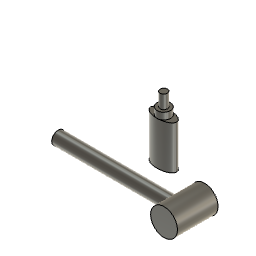
Part3, Assembly of Parts (Autodesk Fusion 360 design; units mm, degrees)
Autodesk Fusion 360 part; units mm, degrees
sketch "Sketch1" plane through (0, 0, 0) normal (0, 0, 1) x (1, 0, 0)
  ellipse E0 centre (0, 0) end of major axis (30.02, 0) minor radius 15.29
  line L0 (-30.02, 0) -> (30.02, 0) construction
  line L1 (0, -15.29) -> (0, 15.29) construction
  dimension "d1" = 60.04
  dimension "d2" = 30.58
  constraint coincident E0 L0.start
  constraint coincident E0 L0.end
  constraint coincident E0 L1.start
  constraint coincident E0 L1.end
  constraint coincident E0.centre origin
  constraint horizontal L0
  measures "d1" distance of E0
extrude "Extrude1" add sketch "Sketch1" along normal blind 99.83 makes body 1
sketch "Sketch2" plane through (0, 0, 0) normal (0, 0, 1) x (1, 0, 0)
  circle A0 centre (0, 0) radius 15.59
  dimension "d5" = 31.18
  constraint coincident A0.centre origin
  measures "d5" diameter of A0
extrude "Extrude3" add sketch "Sketch2" along normal blind 15.57 from surface at 99.83 bodies 1
sketch "Sketch3" plane through (0, 0, 0) normal (0, 0, 1) x (1, 0, 0)
  circle A0 centre (0, 0) radius 8.5
  dimension "d23" = 17
  constraint coincident A0.centre origin
  measures "d23" diameter of A0
extrude "Extrude4" add sketch "Sketch3" along normal blind 31.17 from surface at 115.4 bodies 1
sketch "Sketch5" plane through (0, 0, 0) normal (0, 1, 0) x (1, 0, 0)
  circle A0 centre (0, 0) radius 31
  dimension "d27" = 62
  constraint coincident A0.centre origin
  measures "d27" diameter of A0
extrude "Extrude5" add sketch "Sketch5" along normal blind 93.7 separate body makes body 2
sketch "Sketch6" plane through (0, 0, 0) normal (1, 0, 0) x (0, 1, 0)
  line L0 (0, 0) -> (46.85, 0) construction
  circle A0 centre (46.85, 0) radius 15.01
  dimension "d30" = 46.85
  dimension "d31" = 30.02
  constraint coincident L0.start origin
  constraint horizontal L0
  constraint coincident L0.end A0.centre
  measures "d30" distance of L0.start L0.end
  measures "d31" diameter of A0
extrude "Extrude6" add sketch "Sketch6" against normal blind 264.12 from surface at -26.9565 bodies 2
copy_body "Body->Comp1" bodies 2 removing the originals makes body 3 in component "Component"
copy_body "Body->Comp2" bodies 1 removing the originals makes body 4 in component "Component'"
copy_body "Body->Comp1'" bodies 4 removing the originals makes body 5 in component "Component''"
component "Component" placed x (1, 0, 0) y (0, 1, 0) z (0, 0, 1) at (0, 0, 0)
component "Component'" placed x (1, 0, 0) y (0, 1, 0) z (0, 0, 1) at (0, 0, 0)
component "Component''" placed x (1, 0, 0) y (0, 1, 0) z (0, 0, 1) at (0, 0, 0) in component "Component'"
equation "d1 = container_half_length * 2"
equation "d2 = container_half_width * 2"
equation "d5 = cap_radius * 2"
equation "container_half_width = 15.29 mm"
equation "container_half_length = 30.02 mm"
equation "container_height = 99.83 mm"
equation "cap_radius = 15.59 mm"
equation "cap_height = 15.57 mm"
equation "tip_radius = 8.5 mm"
equation "tip_height = 31.17 mm"
equation "handle_radius = 15.01 mm"
equation "handle_length = 264.12 mm"
equation "sledge_radius = 31 mm"
equation "sledge_length = 93.7 mm"
equation "d20 = container_height"
equation "d21 = cap_height"
equation "d23 = tip_radius * 2"
equation "d24 = cap_height + container_height"
equation "d25 = tip_height"
equation "d27 = sledge_radius * 2"
equation "d28 = sledge_length"
equation "d30 = sledge_length / 2"
equation "d31 = handle_radius * 2"
equation "d32 = sledge_radius / 1.15 * -1"
equation "d33 = handle_length * -1"
